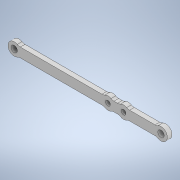
# Autodesk Inventor part: ff
Saved by Autodesk Inventor 2020 (Build 240168000, 168)
## iProperties
Created: 2020-11-09
Part Number: ff
Material: Generic
Document SubType Name: Modeling
Designer: alnwlsn
Density: 1 g/cm^3
Appearance: Default
Author: alnwlsn
Autodesk Inventor part; units mm, degrees
ref_plane "YZ Plane" through (0, 0, 0) normal (1, 0, 0) x (0, 1, 0)
ref_plane "XZ Plane" through (0, 0, 0) normal (0, 1, 0) x (-1, 0, 0)
ref_plane "XY Plane" through (0, 0, 0) normal (0, 0, 1) x (1, 0, 0)
sketch "Sketch1" plane through (0, 0, 0) normal (0, 0, 1) x (1, 0, 0)
  circle A0 centre (0, 0) radius 1
  circle A1 centre (0, 0) radius 2
  line L0 (0, 0) -> (47, 0) construction
  circle A2 centre (47, 0) radius 2
  circle A3 centre (47, 0) radius 1
  line L1 (1, 1.5) -> (46, 1.5)
  line L2 (46, 1.5) -> (46, -1.5)
  line L3 (46, -1.5) -> (1, -1.5)
  line L4 (1, -1.5) -> (1, 1.5)
  line L5 (1, 1.5) -> (46, -1.5) construction
  line L6 (46, 1.5) -> (1, -1.5) construction
  point P0 (23.5, 0)
  point P1 (1.3229, -1.5)
  point P2 (45.6771, -1.5)
  point P3 (45.6771, 1.5)
  point P4 (1.3229, 1.5)
  dimension "d0" = 2
  dimension "d1" = 4
  dimension "d8" = 3
  dimension "d9" = 47
  constraints: 14 end point, 4 centre point, 4 coincident, 3 midpoint, 2 equal radius, 2 horizontal, 2 parallel, 1 perpendicular, 1 tangent
  measures "d0" diameter of A0
  measures "d1" diameter of A1
  measures "d8" distance between parallel lines of L3 L1
  measures "d9" distance of point (0, 0) L0.end
extrude "Extrusion1" add sketch "Sketch1" along normal blind 1.5
fillet "Fillet2" radius 2 4 edges at (1.3229, 1.5, 0.75) (45.6771, 1.5, 0.75) (45.6771, -1.5, 0.75) (1.3229, -1.5, 0.75)
sketch "Sketch3" plane through (0, 0, 1.5) normal (0, 0, 1) x (1, 0, 0)
  line L0 (-12.2, 0) -> (59.2, 0) projected
  circle A0 centre (35, 0) radius 0.75
  circle A1 centre (30, 0) radius 0.75
  circle A2 centre (47, 0) radius 1 projected
  point P0 (0, 0)
  dimension "d11" = 12
  dimension "d12" = 5
  dimension "d13" = 1.5
  constraints: 2 centre point, 2 point on line, 1 equal radius
  measures "d11" distance of A2.centre A0.centre
  measures "d12" distance of A0.centre A1.centre
  measures "d13" diameter of A1
extrude "Extrusion2" cut sketch "Sketch3" against normal through all contours A1 L0 | A0 L0 | L0 A0 | L0 A1
sketch "Sketch4" plane through (0, 0, 1.5) normal (0, 0, 1) x (1, 0, 0)
  circle A0 centre (30, 0) radius 0.75 projected
  circle A1 centre (30, 0) radius 2
  circle A2 centre (35, 0) radius 0.75 projected
  circle A3 centre (35, 0) radius 2
  point P0 (0, 0)
  dimension "d16" = 4
  constraints: 2 centre point, 2 coincident, 1 equal radius
  measures "d16" diameter of A1
extrude "Extrusion3" add sketch "Sketch4" against normal up to surface (1.5 mm away)
fillet "Fillet3" radius 2 8 edges at (28.6771, 1.5, 0.75) (31.3229, 1.5, 0.75) (33.6771, 1.5, 0.75) (36.3229, 1.5, 0.75) (33.6771, -1.5, 0.75) (36.3229, -1.5, 0.75) (28.6771, -1.5, 0.75) (31.3229, -1.5, 0.75)
body "Solid1"
